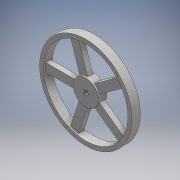
# Autodesk Inventor part: Rueda
Saved by Autodesk Inventor 2016 (Build 200138000, 138)
## iProperties
Created: 2019-03-19
Part Number: Rueda
Material: Genérico
Document SubType Name: Modeling
Designer: FIMCP
Density: 1 g/cm^3
Appearance: Valor por defecto
Author: FIMCP
Autodesk Inventor part; units mm, degrees
ref_plane "YZ Plane" through (0, 0, 0) normal (1, 0, 0) x (0, 1, 0)
ref_plane "XZ Plane" through (0, 0, 0) normal (0, 1, 0) x (-1, 0, 0)
ref_plane "XY Plane" through (0, 0, 0) normal (0, 0, 1) x (1, 0, 0)
sketch "Boceto1" plane through (0, 0, 0) normal (0, 1, 0) x (-1, 0, 0)
  circle A0 centre (0, 0) radius 27.5
  circle A1 centre (0, 0) radius 25
  circle A2 centre (0, 0) radius 7.5
  arc A3 (1, 1.118) -> (1, -1.118) centre (0, 0) ccw
  line L0 (1, 1.118) -> (1, -1.118)
  dimension "d0" = 55
  dimension "d1" = 50
  dimension "d2" = 15
  dimension "d3" = 3
  dimension "d6" = 1
  constraints: 4 centre point, 4 coincident, 2 end point, 2 point on circle
  measures "d0" diameter of A0
  measures "d1" diameter of A1
  measures "d2" diameter of A2
  measures "d3" diameter of A3
  measures "d6" distance from line of L0 point (0, 0)
extrude "Extrusión1" add sketch "Boceto1" along normal mid plane 5
sketch "Boceto2" plane through (0, 0, 0) normal (0, 1, 0) x (-1, 0, 0)
  arc A0 (7.0711, -2.5) -> (7.0711, 2.5) centre (0, 0) ccw
  arc A1 (24.8747, -2.5) -> (24.8747, 2.5) centre (0, 0) ccw
  line L0 (7.0711, 2.5) -> (24.8747, 2.5)
  line L1 (24.8747, -2.5) -> (7.0711, -2.5)
  dimension "d9" = 15
  dimension "d10" = 50
  dimension "d12" = 2.5
  constraints: 4 end point, 4 point on circle, 2 centre point, 2 coincident, 1 horizontal, 1 parallel
  measures "d9" diameter of A0
  measures "d10" diameter of A1
  measures "d12" distance from line of point (0, 0) L1
extrude "Extrusión2" add sketch "Boceto2" along normal mid plane 3
pattern_circular "Patrón circular1" count 5 over 360 about axis through (0, -10, 0) along (0, 1, 0) of "Extrusión2"
